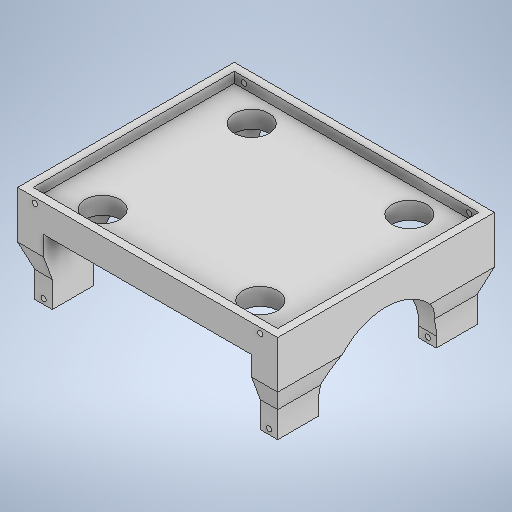
# Autodesk Inventor part: partContainer
Saved by Autodesk Inventor 2025.3 (Build 293356000, 356)
## iProperties
Created: 2025-04-28
Part Number: partContainer
Material: 일반
Document SubType Name: Modeling
Designer: SEON
Density: 1 g/cm^3
Appearance: 기본값
Author: SEON
Autodesk Inventor part; units mm, degrees
ref_plane "YZ Plane" through (0, 0, 0) normal (1, 0, 0) x (0, 1, 0)
ref_plane "XZ Plane" through (0, 0, 0) normal (0, 1, 0) x (-1, 0, 0)
ref_plane "XY Plane" through (0, 0, 0) normal (0, 0, 1) x (1, 0, 0)
sketch "스케치1" plane through (0, 0, 0) normal (0, 0, 1) x (1, 0, 0)
  line L0 (0, 0) -> (15, 0)
  line L1 (15, 0) -> (15, 40)
  line L2 (15, 40) -> (135, 40)
  line L3 (135, 40) -> (135, 0)
  line L4 (135, 0) -> (150, 0)
  line L5 (150, 0) -> (150, 50)
  line L6 (150, 50) -> (0, 50)
  line L7 (0, 50) -> (0, 0)
  line L8 (0, 28.7374) -> (5, 15)
  line L9 (5, 15) -> (5, 0)
  line L10 (75, 50) -> (75, 45.4681)
  line L11 (150, 28.7374) -> (145, 15)
  line L12 (145, 15) -> (145, 0)
  point P0 (145, 0)
  dimension "d0" = 150
  dimension "d1" = 15
  dimension "d2" = 15
  dimension "d3" = 10
  dimension "d4" = 50
  dimension "d7" = 10
  dimension "d8" = 160
  dimension "d9" = 15
  constraints: 26 end point, 7 perpendicular, 4 point on line, 3 symmetric about line, 1 horizontal, 1 midpoint, 1 vertical
  measures "d0" distance between parallel lines of L5 L7
  measures "d1" distance between parallel lines of L7 L1
  measures "d2" distance between parallel lines of L5 L3
  measures "d3" distance between parallel lines of L6 L2
  measures "d4" distance between parallel lines of L0 L6
  measures "d7" distance between parallel lines of L1 L9
  measures "d8" angle of L9 L8
  measures "d9" distance of L8.end L9.end
extrude "돌출1" add sketch "스케치1" along normal blind 125 contours L9 L8 L7 L6 L5 L11 L12 L4 L3 L2 L1 L0
sketch "스케치2" plane through (0, 28.7374, 0) normal (-1, 0, 0) x (0, 0, 1)
  line L0 (0, 21.2626) -> (125, 21.2626) projected
  line L1 (62.5, 21.2626) -> (62.5, 15.0045)
  line L2 (0, 0) -> (0, -13.7374) projected
  line L3 (0, 0) -> (5, -13.7374)
  line L4 (5, -13.7374) -> (5, -28.7374)
  line L5 (0, -28.7374) -> (125, -28.7374) projected
  line L6 (0, 11.2626) -> (0, -28.7374) projected
  line L7 (0, -28.7374) -> (0, 11.2626) projected
  line L8 (0, -13.7374) -> (0, -28.7374) projected
  line L9 (0, 0) -> (0, -13.7374) projected
  line L10 (0, 21.2626) -> (0, 0) projected
  line L11 (0, 0) -> (0, 21.2626) projected
  line L12 (0, -13.7374) -> (0, 0) projected
  line L13 (0, -28.7374) -> (0, -13.7374) projected
  line L14 (125, -28.7374) -> (125, -13.7374) projected
  line L15 (125, -13.7374) -> (125, 0) projected
  line L16 (125, 0) -> (125, 21.2626) projected
  line L17 (125, 21.2626) -> (125, 0) projected
  line L18 (125, 0) -> (125, -13.7374) projected
  line L19 (125, -13.7374) -> (125, -28.7374) projected
  line L20 (125, -28.7374) -> (125, 11.2626) projected
  line L21 (125, 11.2626) -> (125, -28.7374) projected
  line L22 (125, 0) -> (120, -13.7374)
  line L23 (120, -13.7374) -> (120, -28.7374)
  dimension "d10" = 15
  dimension "d11" = 160
  constraints: 10 end point, 3 symmetric about line, 1 midpoint, 1 perpendicular, 1 point on line, 1 vertical
  measures "d10" distance of L3.end L4.end
  measures "d11" angle of L4 L3
extrude "돌출2" cut sketch "스케치2" against normal through all contours L3 L4 L5 L6 L2 | L15 L14 L5 L23 L22
sketch "스케치3" plane through (0, 50, 0) normal (0, 1, 0) x (1, 0, 0)
  line L0 (150, 0) -> (0, 0) projected
  line L1 (0, 0) -> (0, -125) projected
  line L2 (150, -125) -> (0, -125) projected
  line L3 (150, 0) -> (150, -125) projected
  line L4 (4.5, -4.5) -> (145.5, -4.5)
  line L5 (145.5, -4.5) -> (145.5, -120.5)
  line L6 (145.5, -120.5) -> (4.5, -120.5)
  line L7 (4.5, -120.5) -> (4.5, -4.5)
  circle A0 centre (29.5, -19.5) radius 10
  circle A1 centre (29.5, -105.5) radius 10
  circle A2 centre (120.5, -19.5) radius 10
  circle A3 centre (120.5, -105.5) radius 10
  point P0 (0, 0)
  dimension "d14" = 4.5
  dimension "d17" = 20
  dimension "d18" = 15
  dimension "d19" = 25
  dimension "d20" = 25
  dimension "d21" = 15
  constraints: 8 end point, 4 centre point, 3 equal radius, 2 horizontal alignment, 2 vertical alignment, 3 other
  measures "d14" distance between parallel lines of L0 L4
  measures "d17" diameter of A2
  measures "d18" distance from line of L4 A0.centre
  measures "d19" distance from line of L7 A0.centre
  measures "d20" distance from line of L5 A3.centre
  measures "d21" distance from line of L6 A3.centre
extrude "돌출3" add sketch "스케치3" along normal blind 6 contours L3 L2 L1 L0
extrude "돌출4" cut sketch "스케치3" against normal through all contours A0 | A1 | A2 | A3
sketch "스케치5" plane through (0, 0, 0) normal (0, 0, -1) x (-1, 0, 0)
  circle A0 centre (-140, 53) radius 1.5
  line L0 (-135, 0) -> (-145, 0) projected
  line L1 (-150, 56) -> (0, 56) projected
  line L2 (-4.5, 56) -> (-145.5, 56) projected
  line L3 (-75, 56) -> (-75, 53)
  circle A1 centre (-10, 53) radius 1.5
  circle A2 centre (-140, 3) radius 1.5
  circle A3 centre (-10, 3) radius 1.5
  point P0 (0, 0)
  point P1 (-140, 0)
  dimension "d30" = 3
  dimension "d31" = 3
  dimension "d34" = 3
  constraints: 4 centre point, 2 end point, 2 midpoint, 2 symmetric about line, 2 vertical alignment, 1 equal radius, 1 vertical, 2 other
  measures "d30" distance from line of L1 A0.centre
  measures "d31" diameter of A0
  measures "d34" distance from line of L0 A2.centre
extrude "돌출6" cut sketch "스케치5" against normal through all
sketch "스케치6" plane through (0, 28.7374, 0) normal (-1, 0, 0) x (0, 0, 1)
  arc A0 (96.5, -22.7374) -> (28.5, -22.7374) centre (62.5, -22.7374) ccw
  line L0 (5, -28.7374) -> (120, -28.7374) projected
  line L1 (28.5, -22.7374) -> (28.5, -28.7374)
  line L2 (96.5, -28.7374) -> (96.5, -22.7374)
  point P0 (0, -28.7374)
  point P1 (62.5, -28.7374)
  point P2 (99.6652, -28.7374)
  point P3 (25.3348, -28.7374)
  dimension "d35" = 68
  dimension "d38" = 6
  constraints: 4 end point, 2 point on circle, 2 point on line, 2 tangent, 1 centre point, 1 midpoint, 1 perpendicular, 1 vertical, 1 vertical alignment
  measures "d35" diameter of A0
  measures "d38" distance of point (62.5, -28.737) A0.centre
extrude "돌출7" cut sketch "스케치6" against normal through all
equation "\"d10\" = d9"
equation "\"d11\" = d8"
equation "\"d20\" = d19"
equation "\"d21\" = d18"
equation "\"d34\" = d30"
